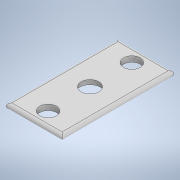
# Autodesk Inventor part: TestBearingTop
Saved by Autodesk Inventor 2022 (Build 260153000, 153)
## iProperties
Created: 2022-03-12
Part Number: TestBearingTop
Material: Generic
Document SubType Name: Modeling
Designer: Jorian Brusind
Density: 1 g/cm^3
Appearance: Default
Author: Jorian Brusind
Autodesk Inventor part; units mm, degrees
ref_plane "YZ Plane" through (0, 0, 0) normal (1, 0, 0) x (0, 1, 0)
ref_plane "XZ Plane" through (0, 0, 0) normal (0, 1, 0) x (-1, 0, 0)
ref_plane "XY Plane" through (0, 0, 0) normal (0, 0, 1) x (1, 0, 0)
sketch "Sketch1" plane through (0, 0, 0) normal (0, 1, 0) x (-1, 0, 0)
  line L0 (-10, -20) -> (10, -20)
  line L1 (10, -20) -> (10, 20)
  line L2 (10, 20) -> (-10, 20)
  line L3 (-10, 20) -> (-10, -20)
  line L4 (-10, -20) -> (10, 20) construction
  line L5 (10, -20) -> (-10, 20) construction
  point P0 (0, 0)
  dimension "d0" = 20
  dimension "d1" = 40
  constraints: 12 end point, 2 midpoint, 2 parallel, 1 horizontal, 1 perpendicular
  measures "d0" distance of L2.end L1.end
  measures "d1" distance of L1.end L0.end
extrude "Extrusion1" add sketch "Sketch1" along normal blind 2
ref_plane "Work Plane1" through (0, 0, 20) normal (1, 0, 0) x (0, 0, -1)
sketch "Sketch3" plane through (0, 0, 20) normal (1, 0, 0) x (0, 0, -1)
  line L0 (40, 0) -> (40, 2) projected
  line L1 (40, 0) -> (20, 0)
  line L2 (40, 0) -> (0, 0) projected
  line L3 (20, 0) -> (20, -3.75)
  line L4 (20, 0) -> (23.75, 0) construction
  arc A0 (23.75, 0) -> (20, 3.75) centre (20, 0) ccw
  line L5 (20, 3.75) -> (20, 0)
  line L6 (20, 0) -> (23.75, 0)
  point P0 (20, 0)
  dimension "d5" = 20
  dimension "d6" = 3.75
  dimension "d7" = 90
  dimension "d8" = 3.75
  constraints: 10 end point, 2 perpendicular, 2 point on circle, 1 centre point, 1 coincident, 1 collinear, 1 horizontal, 1 midpoint, 1 vertical
  measures "d5" distance of L0.start L1.end
  measures "d6" distance of L1.end L3.end
  measures "d7" angle of L3 L4
  measures "d8" radius of A0
revolve "Revolution1" cut sketch "Sketch3" angle 360 about axis through (0, 3.75, 0) along (0, -1, 0)
pattern_of_one "Rectangular Pattern1"
sketch "Sketch4" plane through (0, 2, 0) normal (0, 1, 0) x (1, 0, 0)
  line L0 (-10, -20) -> (10, -20) projected
  line L1 (0, -20) -> (0, -15)
  line L2 (10, 20) -> (-10, 20) projected
  line L3 (0, 20) -> (0, 15)
  circle A0 centre (0, -15) radius 3
  circle A1 centre (0, 15) radius 3
  point P0 (0, 0)
  dimension "d16" = 5
  dimension "d17" = 5
  dimension "d18" = 6
  dimension "d19" = 6
  constraints: 4 end point, 2 centre point, 2 coincident, 2 midpoint, 2 vertical
  measures "d16" distance of L1.start L1.end
  measures "d17" distance of L3.start L3.end
  measures "d18" diameter of A0
  measures "d19" diameter of A1
extrude "Extrusion2" cut sketch "Sketch4" against normal through all
fillet "Fillet1" radius 1 4 edges at (10, 2, 0) (0, 2, 20) (-10, 2, 0) (0, 2, -20)
fillet "Fillet2" radius 1 4 edges at (10, 0, 0) (0, 0, 20) (-10, 0, 0) (0, 0, -20)
body "Solid1"
